Autodesk Inventor part; units mm, degrees
(part 2 of 4)
sketch "Эскиз3" plane through (0, 0, 0) normal (0, 0, -1) x (-1, 0, 0)
  line L0 (-25.3405, 9.161) -> (-25.3405, -5.5092) projected
  line L1 (-25.3405, 9.161) -> (-53, 20.778)
  line L2 (-53, 20.778) -> (-76.2555, 1.8259)
  line L3 (-76.2555, 1.8259) -> (-73.7286, -1.2748)
  line L4 (-73.7286, -1.2748) -> (-53, 15.6179)
  line L5 (-53, 15.6179) -> (-25.3405, 4.0009)
  line L6 (11.1891, 14.3431) -> (11.0924, 14.1698) projected
  arc A0 (11.1891, 14.3431) -> (-16.1963, 14.3431) centre (-2.5036, -3.8906) ccw projected
  arc A1 (-25.3405, 9.161) -> (-16.1963, 14.3431) centre (-40.8164, 47.1281) ccw projected
  line L7 (-25.3405, 9.161) -> (-25.3405, -5.5092) projected
  line L8 (-25.3405, -5.5092) -> (-8.4316, -5.5092) projected
  line L9 (-8.3032, -5.4435) -> (-8.4316, -5.5092) projected
  line L10 (-8.1993, -5.4034) -> (-8.3032, -5.4435) projected
  line L11 (-8.0842, -5.3702) -> (-8.1993, -5.4034) projected
  line L12 (-7.9523, -5.3473) -> (-8.0842, -5.3702) projected
  line L13 (-7.789, -5.3433) -> (-7.9523, -5.3473) projected
  line L14 (-7.444, -5.4468) -> (-7.789, -5.3433) projected
  line L15 (-6.7921, -5.8052) -> (-7.444, -5.4468) projected
  line L16 (-6.1197, -6.1235) -> (-6.7921, -5.8052) projected
  line L17 (-5.8336, -6.3424) -> (-6.1197, -6.1235) projected
  line L18 (-5.7412, -6.4771) -> (-5.8336, -6.3424) projected
  line L19 (-5.6824, -6.5974) -> (-5.7412, -6.4771) projected
  line L20 (-5.6419, -6.7101) -> (-5.6824, -6.5974) projected
  line L21 (-5.6135, -6.8178) -> (-5.6419, -6.7101) projected
  line L22 (-5.5818, -7.0232) -> (-5.6135, -6.8178) projected
  line L23 (-5.5741, -7.2193) -> (-5.5818, -7.0232) projected
  line L24 (-5.5841, -7.4089) -> (-5.5741, -7.2193) projected
  line L25 (-5.6083, -7.5933) -> (-5.5841, -7.4089) projected
  line L26 (-5.691, -7.9502) -> (-5.6083, -7.5933) projected
  line L27 (-5.802, -8.2972) -> (-5.691, -7.9502) projected
  line L28 (-5.8532, -8.6645) -> (-5.802, -8.2972) projected
  line L29 (-5.864, -9.0449) -> (-5.8532, -8.6645) projected
  line L30 (-5.8437, -9.4343) -> (-5.864, -9.0449) projected
  line L31 (-5.7962, -9.8308) -> (-5.8437, -9.4343) projected
  line L32 (-5.7233, -10.2331) -> (-5.7962, -9.8308) projected
  line L33 (-5.6263, -10.6399) -> (-5.7233, -10.2331) projected
  line L34 (-5.5062, -11.0504) -> (-5.6263, -10.6399) projected
  line L35 (-5.3633, -11.4634) -> (-5.5062, -11.0504) projected
  line L36 (-5.1983, -11.8783) -> (-5.3633, -11.4634) projected
  line L37 (-5.0602, -12.1901) -> (-5.1983, -11.8783) projected
  line L38 (-2.9375, -12.5288) -> (-5.0602, -12.1901) projected
  line L39 (-2.7092, -12.2754) -> (-2.9375, -12.5288) projected
  line L40 (-2.4233, -11.9325) -> (-2.7092, -12.2754) projected
  line L41 (-2.159, -11.5843) -> (-2.4233, -11.9325) projected
  line L42 (-1.9171, -11.2317) -> (-2.159, -11.5843) projected
  line L43 (-1.6983, -10.8752) -> (-1.9171, -11.2317) projected
  line L44 (-1.5039, -10.5156) -> (-1.6983, -10.8752) projected
  line L45 (-1.3353, -10.1535) -> (-1.5039, -10.5156) projected
  line L46 (-1.1949, -9.7897) -> (-1.3353, -10.1535) projected
  line L47 (-1.0869, -9.4249) -> (-1.1949, -9.7897) projected
  line L48 (-1.0212, -9.0599) -> (-1.0869, -9.4249) projected
  line L49 (-1.0187, -8.6955) -> (-1.0212, -9.0599) projected
  line L50 (-0.9863, -8.3307) -> (-1.0187, -8.6955) projected
  line L51 (-0.9519, -8.1479) -> (-0.9863, -8.3307) projected
  line L52 (-0.9024, -7.9646) -> (-0.9519, -8.1479) projected
  line L53 (-0.834, -7.7806) -> (-0.9024, -7.9646) projected
  line L54 (-0.74, -7.5953) -> (-0.834, -7.7806) projected
  line L55 (-0.6795, -7.5017) -> (-0.74, -7.5953) projected
  line L56 (-0.6059, -7.4072) -> (-0.6795, -7.5017) projected
  line L57 (-0.5127, -7.3112) -> (-0.6059, -7.4072) projected
  line L58 (-0.3829, -7.2119) -> (-0.5127, -7.3112) projected
  line L59 (-0.0429, -7.0929) -> (-0.3829, -7.2119) projected
  line L60 (0.6951, -6.9997) -> (-0.0429, -7.0929) projected
  line L61 (1.4262, -6.8619) -> (0.6951, -6.9997) projected
  line L62 (1.7863, -6.8709) -> (1.4262, -6.8619) projected
  line L63 (1.9402, -6.9255) -> (1.7863, -6.8709) projected
  line L64 (2.0585, -6.9883) -> (1.9402, -6.9255) projected
  line L65 (2.1575, -7.0556) -> (2.0585, -6.9883) projected
  line L66 (2.2438, -7.1261) -> (2.1575, -7.0556) projected
  line L67 (2.3901, -7.2737) -> (2.2438, -7.1261) projected
  line L68 (2.5117, -7.4278) -> (2.3901, -7.2737) projected
  line L69 (2.615, -7.5871) -> (2.5117, -7.4278) projected
  line L70 (2.7039, -7.7505) -> (2.615, -7.5871) projected
  line L71 (2.8467, -8.0877) -> (2.7039, -7.7505) projected
  line L72 (2.9609, -8.4338) -> (2.8467, -8.0877) projected
  line L73 (3.1354, -8.7611) -> (2.9609, -8.4338) projected
  line L74 (3.3502, -9.0751) -> (3.1354, -8.7611) projected
  line L75 (3.5955, -9.3782) -> (3.3502, -9.0751) projected
  line L76 (3.867, -9.6711) -> (3.5955, -9.3782) projected
  line L77 (4.1624, -9.9537) -> (3.867, -9.6711) projected
  line L78 (4.48, -10.2258) -> (4.1624, -9.9537) projected
  line L79 (4.8185, -10.4872) -> (4.48, -10.2258) projected
  line L80 (5.1768, -10.7375) -> (4.8185, -10.4872) projected
  line L81 (5.5542, -10.9761) -> (5.1768, -10.7375) projected
  line L82 (5.8492, -11.1472) -> (5.5542, -10.9761) projected
  line L83 (7.7656, -10.1735) -> (5.8492, -11.1472) projected
  line L84 (7.8013, -9.8343) -> (7.7656, -10.1735) projected
  line L85 (7.8311, -9.3888) -> (7.8013, -9.8343) projected
  line L86 (7.8403, -8.9518) -> (7.8311, -9.3888) projected
  line L87 (7.8287, -8.5243) -> (7.8403, -8.9518) projected
  line L88 (7.7961, -8.1074) -> (7.8287, -8.5243) projected
  line L89 (7.742, -7.7022) -> (7.7961, -8.1074) projected
  line L90 (7.6656, -7.3102) -> (7.742, -7.7022) projected
  line L91 (7.5654, -6.9333) -> (7.6656, -7.3102) projected
  line L92 (7.4384, -6.5746) -> (7.5654, -6.9333) projected
  line L93 (7.2769, -6.2407) -> (7.4384, -6.5746) projected
  line L94 (7.0647, -5.9445) -> (7.2769, -6.2407) projected
  line L95 (6.8765, -5.6303) -> (7.0647, -5.9445) projected
  line L96 (6.7969, -5.4622) -> (6.8765, -5.6303) projected
  line L97 (6.7292, -5.2848) -> (6.7969, -5.4622) projected
  line L98 (6.6764, -5.0958) -> (6.7292, -5.2848) projected
  line L99 (6.6435, -4.8906) -> (6.6764, -5.0958) projected
  line L100 (6.6374, -4.7793) -> (6.6435, -4.8906) projected
  line L101 (6.6415, -4.6596) -> (6.6374, -4.7793) projected
  line L102 (6.6604, -4.5271) -> (6.6415, -4.6596) projected
  line L103 (6.7071, -4.3705) -> (6.6604, -4.5271) projected
  line L104 (6.9122, -4.0744) -> (6.7071, -4.3705) projected
  line L105 (7.4545, -3.5652) -> (6.9122, -4.0744) projected
  line L106 (7.9649, -3.024) -> (7.4545, -3.5652) projected
  line L107 (8.2615, -2.8196) -> (7.9649, -3.024) projected
  line L108 (8.4182, -2.7733) -> (8.2615, -2.8196) projected
  line L109 (8.5508, -2.7546) -> (8.4182, -2.7733) projected
  line L110 (8.6705, -2.7509) -> (8.5508, -2.7546) projected
  line L111 (8.7817, -2.7571) -> (8.6705, -2.7509) projected
  line L112 (8.9868, -2.7905) -> (8.7817, -2.7571) projected
  line L113 (9.1758, -2.8438) -> (8.9868, -2.7905) projected
  line L114 (9.353, -2.9118) -> (9.1758, -2.8438) projected
  line L115 (9.5209, -2.9918) -> (9.353, -2.9118) projected
  line L116 (9.8347, -3.1808) -> (9.5209, -2.9918) projected
  line L117 (10.1304, -3.3936) -> (9.8347, -3.1808) projected
  line L118 (10.464, -3.5558) -> (10.1304, -3.3936) projected
  line L119 (10.8224, -3.6836) -> (10.464, -3.5558) projected
  line L120 (11.199, -3.7847) -> (10.8224, -3.6836) projected
  line L121 (11.5908, -3.862) -> (11.199, -3.7847) projected
  line L122 (11.9959, -3.917) -> (11.5908, -3.862) projected
  line L123 (12.4128, -3.9505) -> (11.9959, -3.917) projected
  line L124 (12.8403, -3.963) -> (12.4128, -3.9505) projected
  line L125 (13.2773, -3.9548) -> (12.8403, -3.963) projected
  line L126 (13.7228, -3.9261) -> (13.2773, -3.9548) projected
  line L127 (14.0621, -3.891) -> (13.7228, -3.9261) projected
  line L128 (15.0401, -1.9769) -> (14.0621, -3.891) projected
  line L129 (14.8697, -1.6815) -> (15.0401, -1.9769) projected
  line L130 (14.6319, -1.3036) -> (14.8697, -1.6815) projected
  line L131 (14.3824, -0.9447) -> (14.6319, -1.3036) projected
  line L132 (14.1218, -0.6056) -> (14.3824, -0.9447) projected
  line L133 (13.8504, -0.2874) -> (14.1218, -0.6056) projected
  line L134 (13.5684, 0.0086) -> (13.8504, -0.2874) projected
  line L135 (13.2762, 0.2808) -> (13.5684, 0.0086) projected
  line L136 (12.9736, 0.5268) -> (13.2762, 0.2808) projected
  line L137 (12.66, 0.7423) -> (12.9736, 0.5268) projected
  line L138 (12.3332, 0.9175) -> (12.66, 0.7423) projected
  line L139 (11.9874, 1.0325) -> (12.3332, 0.9175) projected
  line L140 (11.6504, 1.1761) -> (11.9874, 1.0325) projected
  line L141 (11.4872, 1.2653) -> (11.6504, 1.1761) projected
  line L142 (11.3282, 1.369) -> (11.4872, 1.2653) projected
  line L143 (11.1743, 1.4909) -> (11.3282, 1.369) projected
  line L144 (11.0271, 1.6375) -> (11.1743, 1.4909) projected
  line L145 (10.9568, 1.724) -> (11.0271, 1.6375) projected
  line L146 (10.8897, 1.8232) -> (10.9568, 1.724) projected
  line L147 (10.8272, 1.9416) -> (10.8897, 1.8232) projected
  line L148 (10.7729, 2.0956) -> (10.8272, 1.9416) projected
  line L149 (10.7647, 2.4558) -> (10.7729, 2.0956) projected
  line L150 (10.9042, 3.1865) -> (10.7647, 2.4558) projected
  line L151 (10.999, 3.9243) -> (10.9042, 3.1865) projected
  line L152 (11.1188, 4.264) -> (10.999, 3.9243) projected
  line L153 (11.2183, 4.3936) -> (11.1188, 4.264) projected
  line L154 (11.3146, 4.4866) -> (11.2183, 4.3936) projected
  line L155 (11.4093, 4.56) -> (11.3146, 4.4866) projected
  line L156 (11.5029, 4.6203) -> (11.4093, 4.56) projected
  line L157 (11.6885, 4.7139) -> (11.5029, 4.6203) projected
  line L158 (11.8727, 4.7818) -> (11.6885, 4.7139) projected
  line L159 (12.056, 4.8309) -> (11.8727, 4.7818) projected
  line L160 (12.2389, 4.8649) -> (12.056, 4.8309) projected
  line L161 (12.6038, 4.8965) -> (12.2389, 4.8649) projected
  line L162 (12.9682, 4.8982) -> (12.6038, 4.8965) projected
  line L163 (13.3334, 4.963) -> (12.9682, 4.8982) projected
  line L164 (13.6984, 5.0703) -> (13.3334, 4.963) projected
  line L165 (14.0625, 5.2099) -> (13.6984, 5.0703) projected
  line L166 (14.425, 5.3776) -> (14.0625, 5.2099) projected
  line L167 (14.785, 5.5713) -> (14.425, 5.3776) projected
  line L168 (15.142, 5.7892) -> (14.785, 5.5713) projected
  line L169 (15.4952, 6.0303) -> (15.142, 5.7892) projected
  line L170 (15.8439, 6.2938) -> (15.4952, 6.0303) projected
  line L171 (16.1875, 6.579) -> (15.8439, 6.2938) projected
  line L172 (16.4414, 6.8067) -> (16.1875, 6.579) projected
  line L173 (16.1075, 8.9301) -> (16.4414, 6.8067) projected
  line L174 (15.796, 9.069) -> (16.1075, 8.9301) projected
  line L175 (15.3815, 9.2349) -> (15.796, 9.069) projected
  line L176 (14.9687, 9.3787) -> (15.3815, 9.2349) projected
  line L177 (14.5586, 9.4998) -> (14.9687, 9.3787) projected
  line L178 (14.1519, 9.5976) -> (14.5586, 9.4998) projected
  line L179 (13.7498, 9.6714) -> (14.1519, 9.5976) projected
  line L180 (13.3534, 9.7199) -> (13.7498, 9.6714) projected
  line L181 (12.964, 9.741) -> (13.3534, 9.7199) projected
  line L182 (12.5837, 9.731) -> (12.964, 9.741) projected
  line L183 (12.2162, 9.6807) -> (12.5837, 9.731) projected
  line L184 (11.8689, 9.5704) -> (12.2162, 9.6807) projected
  line L185 (11.5119, 9.4885) -> (11.8689, 9.5704) projected
  line L186 (11.3274, 9.4648) -> (11.5119, 9.4885) projected
  line L187 (11.1379, 9.4552) -> (11.3274, 9.4648) projected
  line L188 (10.9417, 9.4634) -> (11.1379, 9.4552) projected
  line L189 (10.7364, 9.4955) -> (10.9417, 9.4634) projected
  line L190 (10.6287, 9.5241) -> (10.7364, 9.4955) projected
  line L191 (10.5161, 9.5649) -> (10.6287, 9.5241) projected
  line L192 (10.3959, 9.6239) -> (10.5161, 9.5649) projected
  line L193 (10.2615, 9.7167) -> (10.3959, 9.6239) projected
  line L194 (10.0432, 10.0032) -> (10.2615, 9.7167) projected
  line L195 (9.7265, 10.6764) -> (10.0432, 10.0032) projected
  line L196 (9.3696, 11.329) -> (9.7265, 10.6764) projected
  line L197 (9.2668, 11.6743) -> (9.3696, 11.329) projected
  line L198 (9.2712, 11.8376) -> (9.2668, 11.6743) projected
  line L199 (9.2943, 11.9695) -> (9.2712, 11.8376) projected
  line L200 (9.3278, 12.0845) -> (9.2943, 11.9695) projected
  line L201 (9.3681, 12.1883) -> (9.3278, 12.0845) projected
  line L202 (9.4633, 12.3731) -> (9.3681, 12.1883) projected
  line L203 (9.5723, 12.5363) -> (9.4633, 12.3731) projected
  line L204 (9.6918, 12.6838) -> (9.5723, 12.5363) projected
  line L205 (9.8198, 12.8188) -> (9.6918, 12.6838) projected
  line L206 (10.0964, 13.0589) -> (9.8198, 12.8188) projected
  line L207 (10.3902, 13.2744) -> (10.0964, 13.0589) projected
  line L208 (10.6476, 13.5415) -> (10.3902, 13.2744) projected
  line L209 (10.8798, 13.8428) -> (10.6476, 13.5415) projected
  line L210 (11.0924, 14.1698) -> (10.8798, 13.8428) projected
  circle A2 centre (-8.3767, 1.5633) radius 1.6 projected
  circle A3 centre (2.3455, -2.0471) radius 1.6 projected
  circle A4 centre (5.9559, 8.675) radius 1.6 projected
  circle A5 centre (-4.7663, 12.2855) radius 1.6 projected
  circle A6 centre (-1.2104, 5.1192) radius 2.5 projected
  line L211 (27.6302, -28.9967) -> (27.5395, -29.1586) projected
  line L212 (27.5395, -29.1586) -> (27.3127, -29.5212) projected
  line L213 (27.3127, -29.5212) -> (27.0732, -29.864) projected
  line L214 (27.0732, -29.864) -> (26.8212, -30.1859) projected
  line L215 (26.8212, -30.1859) -> (26.5565, -30.485) projected
  line L216 (26.5565, -30.485) -> (26.279, -30.759) projected
  line L217 (26.279, -30.759) -> (25.9877, -31.0037) projected
  line L218 (25.9877, -31.0037) -> (25.6793, -31.2097) projected
  line L219 (25.6793, -31.2097) -> (25.3462, -31.3574) projected
  line L220 (25.3462, -31.3574) -> (25.0246, -31.5328) projected
  line L221 (25.0246, -31.5328) -> (24.8708, -31.6373) projected
  line L222 (24.8708, -31.6373) -> (24.7225, -31.7559) projected
  line L223 (24.7225, -31.7559) -> (24.5811, -31.892) projected
  line L224 (24.5811, -31.892) -> (24.4487, -32.0522) projected
  line L225 (24.4487, -32.0522) -> (24.3871, -32.145) projected
  line L226 (24.3871, -32.145) -> (24.3298, -32.2502) projected
  line L227 (24.3298, -32.2502) -> (24.279, -32.3741) projected
  line L228 (24.279, -32.3741) -> (24.2398, -32.5327) projected
  line L229 (24.2398, -32.5327) -> (24.2664, -32.892) projected
  line L230 (24.2664, -32.892) -> (24.4757, -33.6058) projected
  line L231 (24.4757, -33.6058) -> (24.6412, -34.3311) projected
  line L232 (24.6412, -34.3311) -> (24.7932, -34.6577) projected
  line L233 (24.7932, -34.6577) -> (24.9047, -34.777) projected
  line L234 (24.9047, -34.777) -> (25.0095, -34.8603) projected
  line L235 (25.0095, -34.8603) -> (25.1108, -34.9243) projected
  line L236 (25.1108, -34.9243) -> (25.2099, -34.9752) projected
  line L237 (25.2099, -34.9752) -> (25.4036, -35.0505) projected
  line L238 (25.4036, -35.0505) -> (25.5935, -35.1004) projected
  line L239 (25.5935, -35.1004) -> (25.7807, -35.1315) projected
  line L240 (25.7807, -35.1315) -> (25.966, -35.1478) projected
  line L241 (25.966, -35.1478) -> (26.3323, -35.144) projected
  line L242 (26.3323, -35.144) -> (26.6951, -35.1105) projected
  line L243 (26.6951, -35.1105) -> (27.0648, -35.1399) projected
  line L244 (27.0648, -35.1399) -> (27.4385, -35.2114) projected
  line L245 (27.4385, -35.2114) -> (27.8144, -35.3153) projected
  line L246 (27.8144, -35.3153) -> (28.1913, -35.4473) projected
  line L247 (28.1913, -35.4473) -> (28.5684, -35.6053) projected
  line L248 (28.5684, -35.6053) -> (28.9447, -35.7878) projected
  line L249 (28.9447, -35.7878) -> (29.3195, -35.9938) projected
  line L250 (29.3195, -35.9938) -> (29.692, -36.2224) projected
  line L251 (29.692, -36.2224) -> (30.0614, -36.4731) projected
  line L252 (30.0614, -36.4731) -> (30.3361, -36.6753) projected
  line L253 (30.3361, -36.6753) -> (30.2085, -38.8211) projected
  line L254 (30.2085, -38.8211) -> (29.9118, -38.9893) projected
  line L255 (29.9118, -38.9893) -> (29.5152, -39.1944) projected
  line L256 (29.5152, -39.1944) -> (29.1183, -39.3773) projected
  line L257 (29.1183, -39.3773) -> (28.7217, -39.5374) projected
  line L258 (28.7217, -39.5374) -> (28.3264, -39.674) projected
  line L259 (28.3264, -39.674) -> (27.9333, -39.7862) projected
  line L260 (27.9333, -39.7862) -> (27.5434, -39.8726) projected
  line L261 (27.5434, -39.8726) -> (27.1579, -39.9312) projected
  line L262 (27.1579, -39.9312) -> (26.7783, -39.958) projected
  line L263 (26.7783, -39.958) -> (26.4077, -39.9433) projected
  line L264 (26.4077, -39.9433) -> (26.0514, -39.867) projected
  line L265 (26.0514, -39.867) -> (25.6882, -39.8199) projected
  line L266 (25.6882, -39.8199) -> (25.5023, -39.814) projected
  line L267 (25.5023, -39.814) -> (25.3126, -39.8228) projected
  line L268 (25.3126, -39.8228) -> (25.1182, -39.8498) projected
  line L269 (25.1182, -39.8498) -> (24.9169, -39.9016) projected
  line L270 (24.9169, -39.9016) -> (24.8125, -39.9405) projected
  line L271 (24.8125, -39.9405) -> (24.7044, -39.9919) projected
  line L272 (24.7044, -39.9919) -> (24.5904, -40.0623) projected
  line L273 (24.5904, -40.0623) -> (24.4655, -40.1675) projected
  line L274 (24.4655, -40.1675) -> (24.2759, -40.4738) projected
  line L275 (24.2759, -40.4738) -> (24.0256, -41.1743) projected
  line L276 (24.0256, -41.1743) -> (23.7332, -41.8584) projected
  line L277 (23.7332, -41.8584) -> (23.6642, -42.2119) projected
  line L278 (23.6642, -42.2119) -> (23.6843, -42.3741) projected
  line L279 (23.6843, -42.3741) -> (23.7201, -42.5031) projected
  line L280 (23.7201, -42.5031) -> (23.7645, -42.6143) projected
  line L281 (23.7645, -42.6143) -> (23.8146, -42.7138) projected
  line L282 (23.8146, -42.7138) -> (23.9271, -42.8885) projected
  line L283 (23.9271, -42.8885) -> (24.0514, -43.0405) projected
  line L284 (24.0514, -43.0405) -> (24.1846, -43.1758) projected
  line L285 (24.1846, -43.1758) -> (24.325, -43.2978) projected
  line L286 (24.325, -43.2978) -> (24.6235, -43.5101) projected
  line L287 (24.6235, -43.5101) -> (24.9367, -43.6962) projected
  line L288 (24.9367, -43.6962) -> (25.2186, -43.9373) projected
  line L289 (25.2186, -43.9373) -> (25.4788, -44.2149) projected
  line L290 (25.4788, -44.2149) -> (25.7219, -44.5198) projected
  line L291 (25.7219, -44.5198) -> (25.9492, -44.8482) projected
  line L292 (25.9492, -44.8482) -> (26.1614, -45.1976) projected
  line L293 (26.1614, -45.1976) -> (26.3585, -45.5664) projected
  line L294 (26.3585, -45.5664) -> (26.5407, -45.9534) projected
  line L295 (26.5407, -45.9534) -> (26.7077, -46.3573) projected
  line L296 (26.7077, -46.3573) -> (26.8592, -46.7773) projected
  line L297 (26.8592, -46.7773) -> (26.9625, -47.1023) projected
  line L298 (26.9625, -47.1023) -> (25.5981, -48.7632) projected
  line L299 (25.5981, -48.7632) -> (25.2592, -48.7249) projected
  line L300 (25.2592, -48.7249) -> (24.8178, -48.6578) projected
  line L301 (24.8178, -48.6578) -> (24.3891, -48.5724) projected
  line L302 (24.3891, -48.5724) -> (23.9742, -48.4688) projected
  line L303 (23.9742, -48.4688) -> (23.5741, -48.347) projected
  line L304 (23.5741, -48.347) -> (23.1901, -48.2067) projected
  line L305 (23.1901, -48.2067) -> (22.8239, -48.0475) projected
  line L306 (22.8239, -48.0475) -> (22.4775, -47.8682) projected
  line L307 (22.4775, -47.8682) -> (22.1548, -47.6668) projected
  line L308 (22.1548, -47.6668) -> (21.8636, -47.4371) projected
  line L309 (21.8636, -47.4371) -> (21.6201, -47.166) projected
  line L310 (21.6201, -47.166) -> (21.354, -46.9143) projected
  line L311 (21.354, -46.9143) -> (21.207, -46.8003) projected
  line L312 (21.207, -46.8003) -> (21.0484, -46.696) projected
  line L313 (21.0484, -46.696) -> (20.8752, -46.6035) projected
  line L314 (20.8752, -46.6035) -> (20.682, -46.5271) projected
  line L315 (20.682, -46.5271) -> (20.5747, -46.4972) projected
  line L316 (20.5747, -46.4972) -> (20.4569, -46.4753) projected
  line L317 (20.4569, -46.4753) -> (20.3234, -46.4652) projected
  line L318 (20.3234, -46.4652) -> (20.1605, -46.4769) projected
  line L319 (20.1605, -46.4769) -> (19.827, -46.6133) projected
  line L320 (19.827, -46.6133) -> (19.2128, -47.0328) projected
  line L321 (19.2128, -47.0328) -> (18.5742, -47.4144) projected
  line L322 (18.5742, -47.4144) -> (18.3105, -47.6599) projected
  line L323 (18.3105, -47.6599) -> (18.2315, -47.8028) projected
  line L324 (18.2315, -47.8028) -> (18.1846, -47.9283) projected
  line L325 (18.1846, -47.9283) -> (18.1551, -48.0444) projected
  line L326 (18.1551, -48.0444) -> (18.1373, -48.1543) projected
  line L327 (18.1373, -48.1543) -> (18.1256, -48.3618) projected
  line L328 (18.1256, -48.3618) -> (18.1368, -48.5578) projected
  line L329 (18.1368, -48.5578) -> (18.165, -48.7455) projected
  line L330 (18.165, -48.7455) -> (18.2068, -48.9267) projected
  line L331 (18.2068, -48.9267) -> (18.3236, -49.2739) projected
  line L332 (18.3236, -49.2739) -> (18.4675, -49.6086) projected
  line L333 (18.4675, -49.6086) -> (18.5539, -49.9694) projected
  line L334 (18.5539, -49.9694) -> (18.6013, -50.3469) projected
  line L335 (18.6013, -50.3469) -> (18.6187, -50.7364) projected
  line L336 (18.6187, -50.7364) -> (18.6096, -51.1357) projected
  line L337 (18.6096, -51.1357) -> (18.5758, -51.5431) projected
  line L338 (18.5758, -51.5431) -> (18.5186, -51.9574) projected
  line L339 (18.5186, -51.9574) -> (18.4385, -52.3775) projected
  line L340 (18.4385, -52.3775) -> (18.3362, -52.8024) projected
  line L341 (18.3362, -52.8024) -> (18.2119, -53.2313) projected
  line L342 (18.2119, -53.2313) -> (18.1045, -53.555) projected
  line L343 (18.1045, -53.555) -> (16.0243, -54.0967) projected
  line L344 (16.0243, -54.0967) -> (15.7727, -53.8665) projected
  line L345 (15.7727, -53.8665) -> (15.455, -53.5527) projected
  line L346 (15.455, -53.5527) -> (15.1584, -53.2317) projected
  line L347 (15.1584, -53.2317) -> (14.8836, -52.904) projected
  line L348 (14.8836, -52.904) -> (14.6315, -52.5703) projected
  line L349 (14.6315, -52.5703) -> (14.4034, -52.2311) projected
  line L350 (14.4034, -52.2311) -> (14.2006, -51.887) projected
  line L351 (14.2006, -51.887) -> (14.0258, -51.5384) projected
  line L352 (14.0258, -51.5384) -> (13.8831, -51.1857) projected
  line L353 (13.8831, -51.1857) -> (13.7825, -50.8287) projected
  line L354 (13.7825, -50.8287) -> (13.7449, -50.4663) projected
  line L355 (13.7449, -50.4663) -> (13.6775, -50.1063) projected
  line L356 (13.6775, -50.1063) -> (13.6256, -49.9276) projected
  line L357 (13.6256, -49.9276) -> (13.5587, -49.75) projected
  line L358 (13.5587, -49.75) -> (13.4729, -49.5734) projected
  line L359 (13.4729, -49.5734) -> (13.3615, -49.398) projected
  line L360 (13.3615, -49.398) -> (13.2922, -49.3107) projected
  line L361 (13.2922, -49.3107) -> (13.2099, -49.2238) projected
  line L362 (13.2099, -49.2238) -> (13.1078, -49.1372) projected
  line L363 (13.1078, -49.1372) -> (12.9691, -49.0509) projected
  line L364 (12.9691, -49.0509) -> (12.6192, -48.9652) projected
  line L365 (12.6192, -48.9652) -> (11.8756, -48.9436) projected
  line L366 (11.8756, -48.9436) -> (11.1347, -48.8769) projected
  line L367 (11.1347, -48.8769) -> (10.7771, -48.9205) projected
  line L368 (10.7771, -48.9205) -> (10.6291, -48.9898) projected
  line L369 (10.6291, -48.9898) -> (10.5175, -49.0637) projected
  line L370 (10.5175, -49.0637) -> (10.4254, -49.1402) projected
  line L371 (10.4254, -49.1402) -> (10.3463, -49.2187) projected
  line L372 (10.3463, -49.2187) -> (10.2149, -49.3797) projected
  line L373 (10.2149, -49.3797) -> (10.1088, -49.5448) projected
  line L374 (10.1088, -49.5448) -> (10.0213, -49.7133) projected
  line L375 (10.0213, -49.7133) -> (9.9486, -49.8845) projected
  line L376 (9.9486, -49.8845) -> (9.8389, -50.234) projected
  line L377 (9.8389, -50.234) -> (9.7587, -50.5894) projected
  line L378 (9.7587, -50.5894) -> (9.6165, -50.932) projected
  line L379 (9.6165, -50.932) -> (9.433, -51.2653) projected
  line L380 (9.433, -51.2653) -> (9.3025, -51.4628) projected
  line L381 (-11.8073, -51.4628) -> (9.3025, -51.4628) projected
  line L382 (-11.8073, -35.0555) -> (-11.8073, -51.4628) projected
  arc A7 (-11.8073, -35.0555) -> (-3.2188, -28.9967) centre (-30.9527, 1.1999) ccw projected
  arc A8 (27.6302, -28.9967) -> (-3.2188, -28.9967) centre (12.2057, -45.7908) ccw projected
  circle A9 centre (19.3845, -32.452) radius 1.6 projected
  circle A10 centre (12.6039, -36.6975) radius 2.5 projected
  circle A11 centre (16.8493, -43.478) radius 1.6 projected
  circle A12 centre (5.8233, -40.9429) radius 1.6 projected
  circle A13 centre (8.3584, -29.9169) radius 1.6 projected
  line L383 (-11.8073, -35.0555) -> (-39.4667, -23.4385)
  line L384 (-39.4667, -23.4385) -> (-62.7223, -42.3906)
  line L385 (-62.7223, -42.3906) -> (-60.1953, -45.4914)
  line L386 (-60.1953, -45.4914) -> (-39.4667, -28.5986)
  line L387 (-39.4667, -28.5986) -> (10.1718, -49.4468)
  line L388 (-11.8073, -35.0555) -> (-11.8073, -40.2156)
  line L389 (-11.8073, -40.2156) -> (10.1718, -49.4468)
  line L390 (-11.8073, -40.2156) -> (10.1718, -49.4468)
  point P0 (0, 0)
  dimension "d4" = 30
  dimension "d5" = 30
  dimension "d6" = 4
  dimension "d11" = 30
  dimension "d12" = 30
  dimension "d13" = 4
  constraints: 26 end point, 4 perpendicular, 4 point on line, 2 parallel, 1 collinear
  measures "d4" distance of L0.start L1.end
  measures "d5" distance of L1.end L2.end
  measures "d6" distance of L2.end L3.end
  measures "d11" distance of L383.start L383.end
  measures "d12" distance of L383.end L384.end
  measures "d13" distance of L384.end L385.end
sketch "Эскиз4" plane through (0, 0, 0) normal (0, 0, -1) x (-1, 0, 0)
  line L0 (11.1891, 14.3431) -> (11.0924, 14.1698) projected
  arc A0 (11.1891, 14.3431) -> (-16.1963, 14.3431) centre (-2.5036, -3.8906) ccw projected
  arc A1 (-25.3405, 9.161) -> (-16.1963, 14.3431) centre (-40.8164, 47.1281) ccw projected
  line L1 (-25.3405, 9.161) -> (-53, 20.778) projected
  line L2 (-53, 20.778) -> (-76.2555, 1.8259) projected
  line L3 (-76.2555, 1.8259) -> (-73.7286, -1.2748) projected
  line L4 (-73.7286, -1.2748) -> (-53, 15.6179) projected
  line L5 (-53, 15.6179) -> (-25.3405, 4.0009) projected
  line L6 (-25.3405, 4.0009) -> (-25.3405, -5.5092) projected
  line L7 (-25.3405, -5.5092) -> (-8.4316, -5.5092) projected
  line L8 (-8.3032, -5.4435) -> (-8.4316, -5.5092) projected
  line L9 (-8.1993, -5.4034) -> (-8.3032, -5.4435) projected
  line L10 (-8.0842, -5.3702) -> (-8.1993, -5.4034) projected
  line L11 (-7.9523, -5.3473) -> (-8.0842, -5.3702) projected
  line L12 (-7.789, -5.3433) -> (-7.9523, -5.3473) projected
  line L13 (-7.444, -5.4468) -> (-7.789, -5.3433) projected
  line L14 (-6.7921, -5.8052) -> (-7.444, -5.4468) projected
  line L15 (-6.1197, -6.1235) -> (-6.7921, -5.8052) projected
  line L16 (-5.8336, -6.3424) -> (-6.1197, -6.1235) projected
  line L17 (-5.7412, -6.4771) -> (-5.8336, -6.3424) projected
  line L18 (-5.6824, -6.5974) -> (-5.7412, -6.4771) projected
  line L19 (-5.6419, -6.7101) -> (-5.6824, -6.5974) projected
  line L20 (-5.6135, -6.8178) -> (-5.6419, -6.7101) projected
  line L21 (-5.5818, -7.0232) -> (-5.6135, -6.8178) projected
  line L22 (-5.5741, -7.2193) -> (-5.5818, -7.0232) projected
  line L23 (-5.5841, -7.4089) -> (-5.5741, -7.2193) projected
  line L24 (-5.6083, -7.5933) -> (-5.5841, -7.4089) projected
  line L25 (-5.691, -7.9502) -> (-5.6083, -7.5933) projected
  line L26 (-5.802, -8.2972) -> (-5.691, -7.9502) projected
  line L27 (-5.8532, -8.6645) -> (-5.802, -8.2972) projected
  line L28 (-5.864, -9.0449) -> (-5.8532, -8.6645) projected
  line L29 (-5.8437, -9.4343) -> (-5.864, -9.0449) projected
  line L30 (-5.7962, -9.8308) -> (-5.8437, -9.4343) projected
  line L31 (-5.7233, -10.2331) -> (-5.7962, -9.8308) projected
  line L32 (-5.6263, -10.6399) -> (-5.7233, -10.2331) projected
  line L33 (-5.5062, -11.0504) -> (-5.6263, -10.6399) projected
  line L34 (-5.3633, -11.4634) -> (-5.5062, -11.0504) projected
  line L35 (-5.1983, -11.8783) -> (-5.3633, -11.4634) projected
  line L36 (-5.0602, -12.1901) -> (-5.1983, -11.8783) projected
  line L37 (-2.9375, -12.5288) -> (-5.0602, -12.1901) projected
  line L38 (-2.7092, -12.2754) -> (-2.9375, -12.5288) projected
  line L39 (-2.4233, -11.9325) -> (-2.7092, -12.2754) projected
  line L40 (-2.159, -11.5843) -> (-2.4233, -11.9325) projected
  line L41 (-1.9171, -11.2317) -> (-2.159, -11.5843) projected
  line L42 (-1.6983, -10.8752) -> (-1.9171, -11.2317) projected
  line L43 (-1.5039, -10.5156) -> (-1.6983, -10.8752) projected
  line L44 (-1.3353, -10.1535) -> (-1.5039, -10.5156) projected
  line L45 (-1.1949, -9.7897) -> (-1.3353, -10.1535) projected
  line L46 (-1.0869, -9.4249) -> (-1.1949, -9.7897) projected
  line L47 (-1.0212, -9.0599) -> (-1.0869, -9.4249) projected
  line L48 (-1.0187, -8.6955) -> (-1.0212, -9.0599) projected
  line L49 (-0.9863, -8.3307) -> (-1.0187, -8.6955) projected
  line L50 (-0.9519, -8.1479) -> (-0.9863, -8.3307) projected
  line L51 (-0.9024, -7.9646) -> (-0.9519, -8.1479) projected
  line L52 (-0.834, -7.7806) -> (-0.9024, -7.9646) projected
  line L53 (-0.74, -7.5953) -> (-0.834, -7.7806) projected
  line L54 (-0.6795, -7.5017) -> (-0.74, -7.5953) projected
  line L55 (-0.6059, -7.4072) -> (-0.6795, -7.5017) projected
  line L56 (-0.5127, -7.3112) -> (-0.6059, -7.4072) projected
  line L57 (-0.3829, -7.2119) -> (-0.5127, -7.3112) projected
  line L58 (-0.0429, -7.0929) -> (-0.3829, -7.2119) projected
  line L59 (0.6951, -6.9997) -> (-0.0429, -7.0929) projected
  line L60 (1.4262, -6.8619) -> (0.6951, -6.9997) projected
  line L61 (1.7863, -6.8709) -> (1.4262, -6.8619) projected
  line L62 (1.9402, -6.9255) -> (1.7863, -6.8709) projected
  line L63 (2.0585, -6.9883) -> (1.9402, -6.9255) projected
  line L64 (2.1575, -7.0556) -> (2.0585, -6.9883) projected
  line L65 (2.2438, -7.1261) -> (2.1575, -7.0556) projected
  line L66 (2.3901, -7.2737) -> (2.2438, -7.1261) projected
  line L67 (2.5117, -7.4278) -> (2.3901, -7.2737) projected
  line L68 (2.615, -7.5871) -> (2.5117, -7.4278) projected
  line L69 (2.7039, -7.7505) -> (2.615, -7.5871) projected
  line L70 (2.8467, -8.0877) -> (2.7039, -7.7505) projected
  line L71 (2.9609, -8.4338) -> (2.8467, -8.0877) projected
  line L72 (3.1354, -8.7611) -> (2.9609, -8.4338) projected
  line L73 (3.3502, -9.0751) -> (3.1354, -8.7611) projected
  line L74 (3.5955, -9.3782) -> (3.3502, -9.0751) projected
  line L75 (3.867, -9.6711) -> (3.5955, -9.3782) projected
  line L76 (4.1624, -9.9537) -> (3.867, -9.6711) projected
  line L77 (4.48, -10.2258) -> (4.1624, -9.9537) projected
  line L78 (4.8185, -10.4872) -> (4.48, -10.2258) projected
  line L79 (5.1768, -10.7375) -> (4.8185, -10.4872) projected
  line L80 (5.5542, -10.9761) -> (5.1768, -10.7375) projected
  line L81 (5.8492, -11.1472) -> (5.5542, -10.9761) projected
  line L82 (7.7656, -10.1735) -> (5.8492, -11.1472) projected
  line L83 (7.8013, -9.8343) -> (7.7656, -10.1735) projected
  line L84 (7.8311, -9.3888) -> (7.8013, -9.8343) projected
  line L85 (7.8403, -8.9518) -> (7.8311, -9.3888) projected
  line L86 (7.8287, -8.5243) -> (7.8403, -8.9518) projected
  line L87 (7.7961, -8.1074) -> (7.8287, -8.5243) projected
  line L88 (7.742, -7.7022) -> (7.7961, -8.1074) projected
  line L89 (7.6656, -7.3102) -> (7.742, -7.7022) projected
  line L90 (7.5654, -6.9333) -> (7.6656, -7.3102) projected
  line L91 (7.4384, -6.5746) -> (7.5654, -6.9333) projected
  line L92 (7.2769, -6.2407) -> (7.4384, -6.5746) projected
  line L93 (7.0647, -5.9445) -> (7.2769, -6.2407) projected
  line L94 (6.8765, -5.6303) -> (7.0647, -5.9445) projected
  line L95 (6.7969, -5.4622) -> (6.8765, -5.6303) projected
  line L96 (6.7292, -5.2848) -> (6.7969, -5.4622) projected
  line L97 (6.6764, -5.0958) -> (6.7292, -5.2848) projected
  line L98 (6.6435, -4.8906) -> (6.6764, -5.0958) projected
  line L99 (6.6374, -4.7793) -> (6.6435, -4.8906) projected
  line L100 (6.6415, -4.6596) -> (6.6374, -4.7793) projected
  line L101 (6.6604, -4.5271) -> (6.6415, -4.6596) projected
  line L102 (6.7071, -4.3705) -> (6.6604, -4.5271) projected
  line L103 (6.9122, -4.0744) -> (6.7071, -4.3705) projected
  line L104 (7.4545, -3.5652) -> (6.9122, -4.0744) projected
  line L105 (7.9649, -3.024) -> (7.4545, -3.5652) projected
  line L106 (8.2615, -2.8196) -> (7.9649, -3.024) projected
  line L107 (8.4182, -2.7733) -> (8.2615, -2.8196) projected
  line L108 (8.5508, -2.7546) -> (8.4182, -2.7733) projected
  line L109 (8.6705, -2.7509) -> (8.5508, -2.7546) projected
  line L110 (8.7817, -2.7571) -> (8.6705, -2.7509) projected
  line L111 (8.9868, -2.7905) -> (8.7817, -2.7571) projected
  line L112 (9.1758, -2.8438) -> (8.9868, -2.7905) projected
  line L113 (9.353, -2.9118) -> (9.1758, -2.8438) projected
  line L114 (9.5209, -2.9918) -> (9.353, -2.9118) projected
  line L115 (9.8347, -3.1808) -> (9.5209, -2.9918) projected
  line L116 (10.1304, -3.3936) -> (9.8347, -3.1808) projected
  line L117 (10.464, -3.5558) -> (10.1304, -3.3936) projected
  line L118 (10.8224, -3.6836) -> (10.464, -3.5558) projected
  line L119 (11.199, -3.7847) -> (10.8224, -3.6836) projected
  line L120 (11.5908, -3.862) -> (11.199, -3.7847) projected
  line L121 (11.9959, -3.917) -> (11.5908, -3.862) projected
  line L122 (12.4128, -3.9505) -> (11.9959, -3.917) projected
  line L123 (12.8403, -3.963) -> (12.4128, -3.9505) projected
  line L124 (13.2773, -3.9548) -> (12.8403, -3.963) projected
  line L125 (13.7228, -3.9261) -> (13.2773, -3.9548) projected
  line L126 (14.0621, -3.891) -> (13.7228, -3.9261) projected
  line L127 (15.0401, -1.9769) -> (14.0621, -3.891) projected
  line L128 (14.8697, -1.6815) -> (15.0401, -1.9769) projected
  line L129 (14.6319, -1.3036) -> (14.8697, -1.6815) projected
  line L130 (14.3824, -0.9447) -> (14.6319, -1.3036) projected
  line L131 (14.1218, -0.6056) -> (14.3824, -0.9447) projected
  line L132 (13.8504, -0.2874) -> (14.1218, -0.6056) projected
  line L133 (13.5684, 0.0086) -> (13.8504, -0.2874) projected
  line L134 (13.2762, 0.2808) -> (13.5684, 0.0086) projected
  line L135 (12.9736, 0.5268) -> (13.2762, 0.2808) projected
  line L136 (12.66, 0.7423) -> (12.9736, 0.5268) projected
  line L137 (12.3332, 0.9175) -> (12.66, 0.7423) projected
  line L138 (11.9874, 1.0325) -> (12.3332, 0.9175) projected
  line L139 (11.6504, 1.1761) -> (11.9874, 1.0325) projected
  line L140 (11.4872, 1.2653) -> (11.6504, 1.1761) projected
  line L141 (11.3282, 1.369) -> (11.4872, 1.2653) projected
  line L142 (11.1743, 1.4909) -> (11.3282, 1.369) projected
  line L143 (11.0271, 1.6375) -> (11.1743, 1.4909) projected
  line L144 (10.9568, 1.724) -> (11.0271, 1.6375) projected
  line L145 (10.8897, 1.8232) -> (10.9568, 1.724) projected
  line L146 (10.8272, 1.9416) -> (10.8897, 1.8232) projected
  line L147 (10.7729, 2.0956) -> (10.8272, 1.9416) projected
  line L148 (10.7647, 2.4558) -> (10.7729, 2.0956) projected
  line L149 (10.9042, 3.1865) -> (10.7647, 2.4558) projected
  line L150 (10.999, 3.9243) -> (10.9042, 3.1865) projected
  line L151 (11.1188, 4.264) -> (10.999, 3.9243) projected
  line L152 (11.2183, 4.3936) -> (11.1188, 4.264) projected
  line L153 (11.3146, 4.4866) -> (11.2183, 4.3936) projected
  line L154 (11.4093, 4.56) -> (11.3146, 4.4866) projected
  line L155 (11.5029, 4.6203) -> (11.4093, 4.56) projected
  line L156 (11.6885, 4.7139) -> (11.5029, 4.6203) projected
  line L157 (11.8727, 4.7818) -> (11.6885, 4.7139) projected
  line L158 (12.056, 4.8309) -> (11.8727, 4.7818) projected
  line L159 (12.2389, 4.8649) -> (12.056, 4.8309) projected
  line L160 (12.6038, 4.8965) -> (12.2389, 4.8649) projected
  line L161 (12.9682, 4.8982) -> (12.6038, 4.8965) projected
  line L162 (13.3334, 4.963) -> (12.9682, 4.8982) projected
  line L163 (13.6984, 5.0703) -> (13.3334, 4.963) projected
  line L164 (14.0625, 5.2099) -> (13.6984, 5.0703) projected
  line L165 (14.425, 5.3776) -> (14.0625, 5.2099) projected
  line L166 (14.785, 5.5713) -> (14.425, 5.3776) projected
  line L167 (15.142, 5.7892) -> (14.785, 5.5713) projected
  line L168 (15.4952, 6.0303) -> (15.142, 5.7892) projected
  line L169 (15.8439, 6.2938) -> (15.4952, 6.0303) projected
  line L170 (16.1875, 6.579) -> (15.8439, 6.2938) projected
  line L171 (16.4414, 6.8067) -> (16.1875, 6.579) projected
  line L172 (16.1075, 8.9301) -> (16.4414, 6.8067) projected
  line L173 (15.796, 9.069) -> (16.1075, 8.9301) projected
  line L174 (15.3815, 9.2349) -> (15.796, 9.069) projected
  line L175 (14.9687, 9.3787) -> (15.3815, 9.2349) projected
  line L176 (14.5586, 9.4998) -> (14.9687, 9.3787) projected
  line L177 (14.1519, 9.5976) -> (14.5586, 9.4998) projected
  line L178 (13.7498, 9.6714) -> (14.1519, 9.5976) projected
  line L179 (13.3534, 9.7199) -> (13.7498, 9.6714) projected
  line L180 (12.964, 9.741) -> (13.3534, 9.7199) projected
  line L181 (12.5837, 9.731) -> (12.964, 9.741) projected
  line L182 (12.2162, 9.6807) -> (12.5837, 9.731) projected
  line L183 (11.8689, 9.5704) -> (12.2162, 9.6807) projected
  line L184 (11.5119, 9.4885) -> (11.8689, 9.5704) projected
  line L185 (11.3274, 9.4648) -> (11.5119, 9.4885) projected
  line L186 (11.1379, 9.4552) -> (11.3274, 9.4648) projected
  line L187 (10.9417, 9.4634) -> (11.1379, 9.4552) projected
  line L188 (10.7364, 9.4955) -> (10.9417, 9.4634) projected
  line L189 (10.6287, 9.5241) -> (10.7364, 9.4955) projected
  line L190 (10.5161, 9.5649) -> (10.6287, 9.5241) projected
  line L191 (10.3959, 9.6239) -> (10.5161, 9.5649) projected
  line L192 (10.2615, 9.7167) -> (10.3959, 9.6239) projected
  line L193 (10.0432, 10.0032) -> (10.2615, 9.7167) projected
  line L194 (9.7265, 10.6764) -> (10.0432, 10.0032) projected
  line L195 (9.3696, 11.329) -> (9.7265, 10.6764) projected
  line L196 (9.2668, 11.6743) -> (9.3696, 11.329) projected
  line L197 (9.2712, 11.8376) -> (9.2668, 11.6743) projected
  line L198 (9.2943, 11.9695) -> (9.2712, 11.8376) projected
  line L199 (9.3278, 12.0845) -> (9.2943, 11.9695) projected
  line L200 (9.3681, 12.1883) -> (9.3278, 12.0845) projected
  line L201 (9.4633, 12.3731) -> (9.3681, 12.1883) projected
  line L202 (9.5723, 12.5363) -> (9.4633, 12.3731) projected
  line L203 (9.6918, 12.6838) -> (9.5723, 12.5363) projected
  line L204 (9.8198, 12.8188) -> (9.6918, 12.6838) projected
  line L205 (10.0964, 13.0589) -> (9.8198, 12.8188) projected
  line L206 (10.3902, 13.2744) -> (10.0964, 13.0589) projected
  line L207 (10.6476, 13.5415) -> (10.3902, 13.2744) projected
  line L208 (10.8798, 13.8428) -> (10.6476, 13.5415) projected
  line L209 (11.0924, 14.1698) -> (10.8798, 13.8428) projected
  circle A2 centre (-8.3767, 1.5633) radius 1.6 projected
  circle A3 centre (2.3455, -2.0471) radius 1.6 projected
  circle A4 centre (5.9559, 8.675) radius 1.6 projected
  circle A5 centre (-4.7663, 12.2855) radius 1.6 projected
  circle A6 centre (-1.2104, 5.1192) radius 2.5 projected
  line L210 (-25.3405, 4.0009) -> (-25.3405, -5.5092) projected
  line L211 (-8.0842, -5.3702) -> (-25.3405, 4.0009)
  point P0 (0, 0)
  constraints: 2 end point
extrude "Выдавливание4" cut sketch "Эскиз4" against normal through all contours L211 L10 L9 L8 L7 L6
extrude "Выдавливание5" add sketch "Эскиз3" against normal up to surface (5 mm away) contours L382 L387 L386 L385 L384 L383
sketch "Эскиз5" plane through (0, 0, 5) normal (0, 0, 1) x (1, 0, 0)
  line L0 (11.8073, -40.2156) -> (-10, -52)
  line L1 (-10, -52) -> (25, -61)
  line L2 (25, -61) -> (11.8073, -40.2156)
  point P0 (0, 0)
  constraints: 6 end point
extrude "Выдавливание6" cut sketch "Эскиз5" against normal through all
mirror "Зеркальное отражение1" about plane through (-26.9625, -47.1023, 0) normal (-0.7726981, -0.6347737, 0)
sketch "Эскиз6" plane through (0, 0, 0) normal (0, 0, -1) x (-1, 0, 0)
  line L0 (25.5981, -48.7632) -> (25.2592, -48.7249) projected
  line L1 (26.8592, -46.7773) -> (26.9625, -47.1023) projected
  line L2 (25.5981, -48.7632) -> (26.9625, -47.1023)
  line L3 (26.9625, -47.1023) -> (64, 11)
  line L4 (64, 11) -> (-98, 3)
  line L5 (-98, 3) -> (-79, -134)
  line L6 (-79, -134) -> (25.5981, -48.7632)
  point P0 (0, 0)
  constraints: 10 end point
extrude "Выдавливание7" cut sketch "Эскиз6" against normal through all